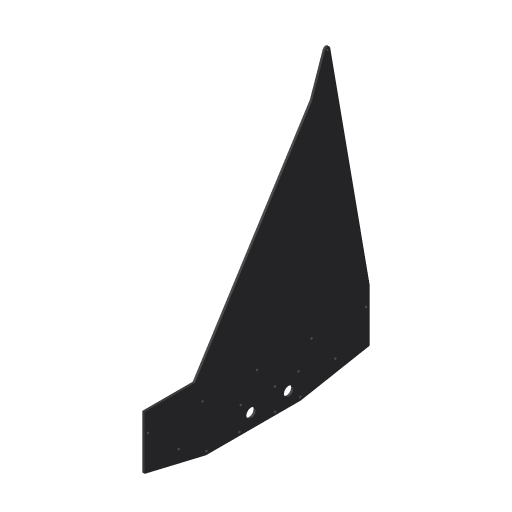
# Autodesk Inventor part: Outside Chassi Plate low 2.0
Saved by Autodesk Inventor 2023 (Build 270158000, 158)
## iProperties
Created: 2022-09-05
Part Number: Outside Chassi Plate low 2.0
Material: Generic
Document SubType Name: Modeling
Designer: deli
Density: 1 g/cm^3
Appearance: Default
Author: deli
Autodesk Inventor part; units mm, degrees
ref_plane "YZ Plane" through (0, 0, 0) normal (1, 0, 0) x (0, 1, 0)
ref_plane "XZ Plane" through (0, 0, 0) normal (0, 1, 0) x (-1, 0, 0)
ref_plane "XY Plane" through (0, 0, 0) normal (0, 0, 1) x (1, 0, 0)
sketch "Sketch1" plane through (0, 0, 0) normal (1, 0, 0) x (0, 1, 0)
  line L0 (-213.0456, 459.9281) -> (-291.6852, 459.9281)
  line L1 (-291.6852, 459.9281) -> (-312.9107, 370.4439)
  line L2 (-215.2523, 129.9281) -> (-293.8918, 129.9281)
  circle A0 centre (-285.0456, 409.9281) radius 2
  circle A1 centre (-285.0456, 409.9281) radius 48 construction
  arc A2 (-273.131, 409.2041) -> (-296.9481, 410.8302) centre (-285.0456, 409.9281) ccw construction
  circle A3 centre (-285.0456, 179.9281) radius 48 construction
  arc A4 (-296.901, 178.5379) -> (-273.1614, 181.0447) centre (-285.0456, 179.9281) ccw construction
  circle A5 centre (-285.0456, 179.9281) radius 2
  circle A6 centre (-292.2956, 303.7379) radius 7
  circle A7 centre (-292.2956, 248.5853) radius 7
  circle A8 centre (-292.2956, 303.7379) radius 18.75 construction
  circle A9 centre (-292.2956, 248.5853) radius 18.75 construction
  arc A10 (-304.9916, 304.7001) -> (-279.5867, 302.9656) centre (-292.2956, 303.7379) ccw construction
  arc A11 (-279.6191, 249.7764) -> (-304.9414, 247.1024) centre (-292.2956, 248.5853) ccw construction
  line L3 (-273.131, 409.2041) -> (-279.5867, 302.9656) construction
  line L4 (-304.9916, 304.7001) -> (-296.9481, 410.8302) construction
  line L5 (-279.6191, 249.7764) -> (-273.1614, 181.0447) construction
  line L6 (-296.901, 178.5379) -> (-304.9414, 247.1024) construction
  circle A12 centre (-276.1617, 268.6542) radius 2
  circle A13 centre (-308.4296, 268.6542) radius 2
  circle A14 centre (-308.0456, 320.8406) radius 2
  circle A15 centre (-308.0456, 231.4827) radius 2
  circle A16 centre (-274.1266, 234.0785) radius 2
  circle A17 centre (-242.0456, 454.9281) radius 2
  arc A18 (-313.0456, 229.9036) -> (-313.0456, 229.9036) centre (-290.2956, 229.9036) ccw
  line L7 (-313.0456, 231.4827) -> (-313.0456, 229.9036)
  arc A19 (-312.9107, 370.4439) -> (-313.0456, 369.2899) centre (-308.0456, 369.2899) ccw
  line L8 (-313.0456, 369.2899) -> (-313.0456, 229.9036)
  line L9 (-293.8918, 129.9281) -> (-312.9582, 230.5519)
  circle A20 centre (-274.6149, 318.8361) radius 2
  arc A21 (-313.0456, 231.4827) -> (-312.9582, 230.5519) centre (-308.0456, 231.4827) ccw
  circle A22 centre (-242.0456, 214.9281) radius 2
  line L10 (-213.0456, 459.9281) -> (-213.0456, 386.3041)
  circle A23 centre (-242.0456, 374.9281) radius 2
  circle A24 centre (-242.0456, 294.9281) radius 2
  circle A25 centre (-308.0456, 369.2899) radius 2
  circle A26 centre (-242.0456, 134.9281) radius 2
  line L11 (-225.2933, 129.9281) -> (161.5427, 129.9281)
  line L12 (161.5427, 129.9281) -> (161.5427, 149.9281)
  line L13 (161.5427, 149.9281) -> (-213.0456, 386.3041)
  line L14 (-193.9002, 374.2228) -> (-204.5734, 357.3088)
  line L15 (-204.5734, 357.3088) -> (49.1363, 197.2107)
  line L16 (49.1363, 197.2107) -> (59.8095, 214.1247)
  circle A27 centre (-201.0456, 382.5748) radius 4.125
  circle A28 centre (113.5544, 184.0531) radius 4.125 construction
  line L17 (31.7149, 208.2041) -> (30.6476, 206.5127)
  line L18 (30.6476, 206.5127) -> (48.4072, 195.3059)
  line L19 (48.4072, 195.3059) -> (49.4745, 196.9973)
  line L20 (49.4745, 196.9973) -> (49.1363, 197.2107)
  line L21 (49.1363, 197.2107) -> (6.679, 129.9281)
  circle A29 centre (-186.5513, 357.7609) radius 1.5
  circle A30 centre (-72.382, 285.7168) radius 1.5
  circle A31 centre (41.7874, 213.6726) radius 1.5
  circle A32 centre (112.9507, 191.5288) radius 1.6
  circle A33 centre (112.9507, 191.5288) radius 6 construction
  arc A34 (113.6414, 187.5889) -> (114.2571, 195.3094) centre (112.9507, 191.5288) ccw
  line L22 (59.8095, 214.1247) -> (114.2571, 195.3094)
  line L23 (-215.2523, 129.9281) -> (113.6414, 187.5889)
  point P0 (0, 0)
  point P1 (-200.6317, 378.4706)
  point P2 (-204.9284, 381.1819)
  point P3 (104.4225, 185.9726)
  dimension "d44" = 4
  dimension "d46" = 96
  dimension "d47" = 23.8732
  dimension "d48" = 96
  dimension "d49" = 4
  dimension "d51" = 23.8732
  dimension "d54" = 50
  dimension "d55" = 50
  dimension "d58" = 14
  dimension "d59" = 14
  dimension "d60" = 37.5
  dimension "d61" = 37.5
  dimension "d62" = 25.4648
  dimension "d63" = 25.4648
  dimension "d64" = 179.143
  dimension "d65" = 179.143
  dimension "d66" = 178.679
  dimension "d67" = 178.679
  dimension "d68" = 106.4344
  dimension "d70" = 69.0344
  dimension "d74" = 4
  dimension "d75" = 4
  dimension "d77" = 4
  dimension "d78" = 4
  dimension "d94" = 2.5
  dimension "d95" = 2.5
  dimension "d97" = 2.5
  dimension "d103" = 4
  dimension "d120" = 4
  dimension "d124" = 28
  dimension "d125" = 20.75
  dimension "d127" = 20.75
  dimension "d142" = 4
  dimension "d143" = 2.5
  dimension "d144" = 4
  dimension "d145" = 4
  dimension "d146" = 18
  dimension "d147" = 18
  dimension "d148" = 5
  dimension "d149" = 5
  dimension "d153" = 4
  dimension "d166" = 5
  dimension "d218" = 0
  dimension "d235" = 29
  dimension "d244" = 24
  dimension "d246" = 78.6395
  dimension "d247" = 78.6395
  dimension "d258" = 5
  dimension "d259" = 5
  dimension "d260" = 4
  dimension "d261" = 4
  dimension "d262" = 4
  dimension "d264" = 5
  dimension "d266" = 29
  dimension "d267" = 29
  dimension "d268" = 80
  dimension "d269" = 80
  dimension "d270" = 80
  dimension "d271" = 0
  dimension "d272" = 48.4494
  dimension "d277" = 5
  dimension "d279" = 20
  dimension "d296" = 29
  dimension "d297" = 20
  constraints: 48 end point, 35 centre point, 17 point on circle, 16 tangent, 8 perpendicular, 7 coincident, 5 point on line, 4 concentric, 4 equal radius, 4 vertical, 2 parallel, 1 collinear, 1 horizontal
  measures "d44" diameter of A0
  measures "d46" diameter of A1
  measures "d47" diameter of A2
  measures "d48" diameter of A3
  measures "d49" diameter of A5
  measures "d51" diameter of A4
  measures "d54" distance from line of A0.centre L0
  measures "d55" distance from line of L2 A5.centre
  measures "d58" diameter of A6
  measures "d59" diameter of A7
  measures "d60" diameter of A8
  measures "d61" diameter of A9
  measures "d62" diameter of A10
  measures "d63" diameter of A11
  measures "d68" distance of L3.start L3.end
  measures "d70" distance of L5.start L5.end
  measures "d74" diameter of A14
  measures "d75" diameter of A13
  measures "d77" diameter of A12
  measures "d78" diameter of A16
  measures "d103" diameter of A17
  measures "d120" diameter of A15
  measures "d124" distance from line of A0.centre L7
  measures "d125" distance from line of L7 A6.centre
  measures "d127" distance from line of L7 A7.centre
  measures "d142" distance from line of L5 A16.centre
  measures "d144" distance from line of L3 A20.centre
  measures "d145" diameter of A20
  measures "d146" distance from line of A0.centre L1
  measures "d147" distance from line of L9 A3.centre
  measures "d148" radius of A19
  measures "d149" radius of A21
  measures "d153" diameter of A22
  measures "d166" distance from line of L8 A14.centre
  measures "d218" horizontal distance of A0.centre A5.centre
  measures "d235" distance from line of L10 A17.centre
  measures "d244" distance edge to line of A1 L10
  measures "d246" distance of L2.start L2.end
  measures "d247" distance of L0.start L0.end
  measures "d260" diameter of A23
  measures "d261" diameter of A24
  measures "d262" diameter of A25
  measures "d264" distance from line of L8 A25.centre
  measures "d266" distance from line of L10 A23.centre
  measures "d267" distance from line of L10 A24.centre
  measures "d268" distance of A23.centre A17.centre
  measures "d269" distance of A24.centre A23.centre
  measures "d270" distance of A22.centre A24.centre
  measures "d271" distance of A25.centre A19.centre
  measures "d272" distance of A14.centre A25.centre
  measures "d277" distance from line of L2 A26.centre
  measures "d279" distance of L12.end L11.end
  measures "d296" distance from line of L10 A22.centre
  measures "d297" distance of L14.start L14.end
extrude "Extrusion1" add sketch "Sketch1" along normal blind 3.175 contours L10 L13 A27 L14 L15 L17 L18 L21 L23 L2 L9 A18 A7 A21 L8 A19 L1 L0 | L13 A27 | L13 L16 L15 L14 | A18 A7 L9 A21 | L22 A34 L23 L13 | L13 L23 L21 L18 L19 L20 L16 | L21 L18 L17 L15 | L20 L19 L18 L21 picked at (-202.3674, 379.3774)
thread "Thread1" size "M3x0.5" class "6H" standard "ANSI Metric M Profile" full length
thread "Thread2" size "M3x0.5" class "6H" standard "ANSI Metric M Profile" full length
thread "Thread3" size "M3x0.5" class "6H" standard "ANSI Metric M Profile" full length
fillet "Fillet1" radius 2 2 edges at (1.5875, 59.8095, 214.1247) (1.5875, -213.0456, 386.3041)
body "Solid1"
